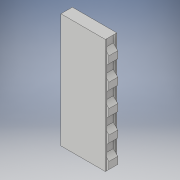
# Autodesk Inventor part: door (left side) 2nd map
Saved by Autodesk Inventor 2017 (Build 210142000, 142)
## iProperties
Created: 2018-05-21
Part Number: door (left side) 2nd map
Material: Generic
Document SubType Name: Modeling
Designer: braxtonwright
Density: 1 g/cm^3
Appearance: Default
Author: braxtonwright
Autodesk Inventor part; units mm, degrees
ref_plane "YZ Plane" through (0, 0, 0) normal (1, 0, 0) x (0, 1, 0)
ref_plane "XZ Plane" through (0, 0, 0) normal (0, 1, 0) x (-1, 0, 0)
ref_plane "XY Plane" through (0, 0, 0) normal (0, 0, 1) x (1, 0, 0)
sketch "Sketch1" plane through (0, 0, 0) normal (0, 0, 1) x (1, 0, 0)
  line L0 (0, 0) -> (88.9, 0)
  line L1 (88.9, 0) -> (88.9, 228.6)
  line L2 (88.9, 228.6) -> (0, 228.6)
  line L3 (0, 228.6) -> (0, 0)
  dimension "d0" = 88.9
  dimension "d1" = 228.6
  constraints: 8 end point, 2 parallel, 1 horizontal, 1 perpendicular
  measures "d0" distance of L2.end L1.end
  measures "d1" distance of L0.end L1.end
extrude "door" add sketch "Sketch1" along normal mid plane 22.86
sketch "Sketch2" plane through (0, 0, 0) normal (0, 0, 1) x (1, 0, 0)
  line L0 (88.9, 228.6) -> (0, 228.6) projected
  line L1 (88.9, 0) -> (0, 0) projected
  line L2 (88.9, 228.6) -> (84.4099, 224.1099)
  line L3 (84.4099, 224.1099) -> (84.4099, 210.2301)
  line L4 (84.4099, 210.2301) -> (88.9, 205.74)
  line L5 (88.9, 205.74) -> (93.3901, 201.2499)
  line L6 (93.3901, 201.2499) -> (93.3901, 187.3701)
  line L7 (93.3901, 187.3701) -> (88.9, 182.88)
  line L8 (88.9, 182.88) -> (84.4099, 178.3899)
  line L9 (84.4099, 178.3899) -> (84.4099, 164.5101)
  line L10 (84.4099, 164.5101) -> (88.9, 160.02)
  line L11 (88.9, 160.02) -> (93.3901, 155.5299)
  line L12 (93.3901, 155.5299) -> (93.3901, 141.6501)
  line L13 (93.3901, 141.6501) -> (88.9, 137.16)
  line L14 (88.9, 137.16) -> (84.4099, 132.6699)
  line L15 (84.4099, 132.6699) -> (84.4099, 118.7901)
  line L16 (84.4099, 118.7901) -> (88.9, 114.3)
  line L17 (88.9, 114.3) -> (93.3901, 109.8099)
  line L18 (93.3901, 109.8099) -> (93.3901, 95.9301)
  line L19 (93.3901, 95.9301) -> (88.9, 91.44)
  line L20 (88.9, 91.44) -> (84.4099, 86.9499)
  line L21 (84.4099, 86.9499) -> (84.4099, 73.0701)
  line L22 (84.4099, 73.0701) -> (88.9, 68.58)
  line L23 (88.9, 68.58) -> (93.3901, 64.0899)
  line L24 (93.3901, 64.0899) -> (93.3901, 50.2101)
  line L25 (93.3901, 50.2101) -> (88.9, 45.72)
  line L26 (88.9, 45.72) -> (84.4099, 41.2299)
  line L27 (84.4099, 41.2299) -> (84.4099, 27.3501)
  line L28 (84.4099, 27.3501) -> (88.9, 22.86)
  line L29 (88.9, 22.86) -> (93.3901, 18.3699)
  line L30 (93.3901, 18.3699) -> (93.3901, 4.4901)
  line L31 (93.3901, 4.4901) -> (88.9, 0)
  line L32 (88.9, 0) -> (88.9, 22.86)
  line L33 (88.9, 22.86) -> (88.9, 45.72)
  line L34 (88.9, 45.72) -> (88.9, 68.58)
  line L35 (88.9, 68.58) -> (88.9, 91.44)
  line L36 (88.9, 91.44) -> (88.9, 114.3)
  line L37 (88.9, 114.3) -> (88.9, 137.16)
  line L38 (88.9, 137.16) -> (88.9, 160.02)
  line L39 (88.9, 160.02) -> (88.9, 182.88)
  line L40 (88.9, 182.88) -> (88.9, 205.74)
  line L41 (88.9, 205.74) -> (88.9, 228.6)
  point P0 (84.4099, 217.17)
  point P1 (93.3901, 194.31)
  point P2 (84.4099, 171.45)
  point P3 (93.3901, 148.59)
  point P4 (84.4099, 125.73)
  point P5 (93.3901, 102.87)
  point P6 (84.4099, 80.01)
  point P7 (93.3901, 57.15)
  point P8 (84.4099, 34.29)
  dimension "d7" = 228.6
  dimension "d23" = 6.35
  dimension "d24" = 228.6
  dimension "d25" = 11.43
  dimension "d26" = 11.43
  dimension "d27" = 11.43
  dimension "d28" = 11.43
  dimension "d29" = 11.43
  dimension "d30" = 11.43
  dimension "d31" = 11.43
  dimension "d32" = 11.43
  dimension "d34" = 45
  dimension "d35" = 45
  constraints: 80 end point, 14 point on line, 11 equal length, 9 collinear, 9 midpoint, 8 perpendicular, 6 vertical
  measures "d7" distance of L0.end L1.end
  measures "d23" distance of L0.start L2.end
  measures "d24" distance of L1.start L0.start
  measures "d25" vertical distance of point (93.39, 194.31) L40.end
  measures "d26" vertical distance of L39.end point (84.41, 171.45)
  measures "d27" vertical distance of L39.start point (93.39, 148.59)
  measures "d28" vertical distance of point (84.41, 125.73) L13.end
  measures "d29" vertical distance of point (93.39, 102.87) L37.start
  measures "d30" vertical distance of point (84.41, 80.01) L35.end
  measures "d31" vertical distance of point (93.39, 57.15) L34.end
  measures "d32" vertical distance of point (84.41, 34.29) L25.end
  measures "d34" angle of L2 L41
  measures "d35" angle of L41 L4
extrude "teeth cut" cut sketch "Sketch2" along normal mid plane 17.78 contours L41 L4 L3 L2 | L33 L28 L27 L26 | L35 L22 L21 L20 | L37 L16 L15 L14 | L39 L10 L9 L8
extrude "teeth make" add sketch "Sketch2" along normal mid plane 17.78 contours L29 L30 L31 L32 | L23 L24 L25 L34 | L17 L18 L19 L36 | L11 L12 L13 L38 | L5 L6 L7 L40
equation "\"d25\" = d33"
equation "\"d26\" = d33"
equation "\"d27\" = d33"
equation "\"d28\" = d33"
equation "\"d29\" = d33"
equation "\"d30\" = d33"
equation "\"d31\" = d33"
equation "\"d32\" = d33"
equation "\"d21\" = d19"
equation "\"d33\" = 0.05 * d24"
equation "\"d19\" = 17.78"
body "Solid1"
